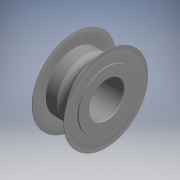
# Autodesk Inventor part: W 619/3-2Z_PART1
Saved by Autodesk Inventor 2017.3 (Build 213256000, 256)
## iProperties
Part Number: W 619/3-2Z_PART1
Material: Generic
Catalog Web Link: www.cadenas.de
Description: -Deep groove ball bearings
Vendor: SKF
Document SubType Name: Modeling
Designer: partserver
Manufacturer: SKF
Mass: 0.038513 g
Surface Area: 1.9413 cm^2
Volume: 0.038513 cm^3
Density: 1 g/cm^3
Appearance: PSOLRGB-175-175-175
Category: PARTsolutions
Company: SKF
Title: W 619/3-2Z_PART1
Author: Cadenas PARTsolutions
Comments: Deep groove ball bearings
PSOL_IDENT_0: {$CADENAS_DATA\23d-libs\skf\bearings_units_and_housings\ball_bearings\deep_groove_ball_bearings\bb1_
PSOL_IDENT_1: 001_101.prj},199 {VTYP=3D},{NB=W 619/3-2Z_PART1},{LINA=W 619/3-2Z_PART1},{NN=BB1_001_101_PART1},{NOP
PSOL_IDENT_2: RJ=TRUE},{DATE=19.12.2019 14:34:47},{GEOMDATE=18.12.2019 13:53:11},{VERSION=},{LINEID=17690},{WBVAR=
PSOL_IDENT_3: },{WBNUMERIC=}  {NB=W 619/3-2Z_PART1},{LINA=W 619/3-2Z_PART1},{KT=DUMMY},{PRODUCTID=1010476193},{DES
PSOL_IDENT_4: IGNATION=W 619/3-2Z},{DD=3.000},{D=8.000},{B=3.000},{C=0.000},{DD1=5.00},{DD2=0.00},{D1=0.00},{D2=7.
PSOL_IDENT_5: 40},{D3=0.000},{D4=0.000},{HH=MIN},{BB=0.000},{FF=0.00},{R0MAX=MIN},{R0=MIN},{R12=0.10},{PITCH=5.90}
PSOL_IDENT_6: ,{DW=1.200},{DDAMIN=3.800},{DDAMAX=4.900},{DDBMIN=MIN},{DDBMAX=MIN},{DBMIN=MIN},{DAMAX=7.500},{BBAMI
PSOL_IDENT_7: N=MIN},{CAMAX=MIN},{RAMAX=0.100},{LOAD1=0.225},{LOAD2=0.072},{LOAD3=0.003},{SPEED1=150000},{SPEED2=7
PSOL_IDENT_8: 5000},{KR=0.025},{F0=7.200},{Z=7},{II=1},{MASS=0.001},{BEARING=W 619/3-2Z},{RING=},{HELP=0.648},{HEL
PSOL_IDENT_9: P2=0.300},{DD1ALG=2.500},{YALG=2.500},{PITCH1=5.900},{DW1=1.200},{YALG1=3.352},{HALG1=0.648},{SH=2.5
PSOL_IDENT_10: 00},{CU=0.360},{DESIGN=dgbbw2z},{HALG=1},{B1=0},{SHIELDHELP=2}
NB: W 619/3-2Z_PART1
NT: Deep groove ball bearings
NBSYN: $DESIGNATION._PART1
LINA: W 619/3-2Z_PART1
CATALOG: SKF
SUPPLIER: SKF
ARTICLENO: W 619/3-2Z_PART1
BOMINFO: W 619/3-2Z_PART1
CREATOR: CADENAS GmbH
Autodesk Inventor part; units mm, degrees
ref_plane "YZ Plane" through (0, 0, 0) normal (1, 0, 0) x (0, 1, 0)
ref_plane "XZ Plane" through (0, 0, 0) normal (0, 1, 0) x (-1, 0, 0)
ref_plane "XY Plane" through (0, 0, 0) normal (0, 0, 1) x (1, 0, 0)
sketch "Sketch_17" plane through (0, 0, 0) normal (0, 0, 1) x (1, 0, 0)
  line L0 (50, 0) -> (-50, 0)
  line L1 (0, 2.48) -> (0, 1.6)
  arc A0 (0, 1.6) -> (0.1, 1.5) centre (0.1, 1.6) ccw
  line L2 (0.1, 1.5) -> (2.9, 1.5)
  arc A1 (2.9, 1.5) -> (3, 1.6) centre (2.9, 1.6) ccw
  line L3 (3, 1.6) -> (3, 2.48)
  arc A2 (3, 2.48) -> (2.98, 2.5) centre (2.98, 2.48) ccw
  line L4 (2.98, 2.5) -> (1.8969, 2.5)
  arc A3 (1.1031, 2.5) -> (1.8969, 2.5) centre (1.5, 2.95) ccw
  line L5 (1.1031, 2.5) -> (0.02, 2.5)
  arc A4 (0.02, 2.5) -> (0, 2.48) centre (0.02, 2.48) ccw
  constraints: 12 end point, 10 point on circle, 5 centre point
revolve "Revolution1" add sketch "Sketch_17" angle 360 about axis through (50, 0, 0) along (1, 0, 0)
sketch "Sketch_20" plane through (0, 0, 0) normal (0, 0, 1) x (1, 0, 0)
  line L0 (50, 0) -> (-50, 0)
  line L1 (0.09, 3.7) -> (0.105, 3.3975)
  line L2 (0.105, 3.3975) -> (0.09, 3.095)
  line L3 (0.09, 3.095) -> (0.09, 2.49)
  line L4 (0.09, 2.49) -> (0.12, 2.49)
  line L5 (0.12, 2.49) -> (0.15, 3.095)
  line L6 (0.15, 3.095) -> (0.15, 3.3975)
  line L7 (0.15, 3.3975) -> (0.12, 3.7)
  line L8 (0.12, 3.7) -> (0.09, 3.7)
  constraints: 18 end point
revolve "Revolution2" add sketch "Sketch_20" angle 360 about axis through (50, 0, 0) along (1, 0, 0)
sketch "Sketch_21" plane through (0, 0, 0) normal (0, 0, 1) x (1, 0, 0)
  line L0 (50, 0) -> (-50, 0)
  line L1 (2.85, 3.3975) -> (2.85, 3.095)
  line L2 (2.85, 3.095) -> (2.88, 2.49)
  line L3 (2.88, 2.49) -> (2.91, 2.49)
  line L4 (2.91, 2.49) -> (2.91, 3.095)
  line L5 (2.91, 3.095) -> (2.895, 3.3975)
  line L6 (2.895, 3.3975) -> (2.91, 3.7)
  line L7 (2.91, 3.7) -> (2.88, 3.7)
  line L8 (2.88, 3.7) -> (2.85, 3.3975)
  constraints: 18 end point
revolve "Revolution3" add sketch "Sketch_21" angle 360 about axis through (50, 0, 0) along (1, 0, 0)
body "Solid1"
